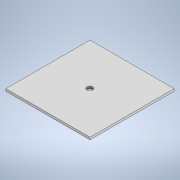
# Autodesk Inventor part: Base
Saved by Autodesk Inventor 2020 (Build 240168000, 168)
## iProperties
Created: 2019-09-27
Part Number: Base
Material: Genérico
Document SubType Name: Modeling
Designer: Java9
Density: 1 g/cm^3
Appearance: Valor por defecto
Author: Java9
Autodesk Inventor part; units mm, degrees
ref_plane "YZ Plane" through (0, 0, 0) normal (1, 0, 0) x (0, 1, 0)
ref_plane "XZ Plane" through (0, 0, 0) normal (0, 1, 0) x (-1, 0, 0)
ref_plane "XY Plane" through (0, 0, 0) normal (0, 0, 1) x (1, 0, 0)
sketch "Boceto1" plane through (0, 0, 0) normal (0, 0, 1) x (1, 0, 0)
  line L0 (0, 0) -> (450, 0)
  line L1 (450, 0) -> (450, 12.7)
  line L2 (450, 12.7) -> (0, 12.7)
  line L3 (0, 12.7) -> (0, 0)
  dimension "d0" = 450
  dimension "d1" = 12.7
  constraints: 8 end point, 2 perpendicular, 1 horizontal, 1 parallel
  measures "d0" distance of L0.start L0.end
  measures "d1" distance of L0.end L1.end
extrude "Extrusión1" add sketch "Boceto1" along normal blind 450
sketch "Boceto2" plane through (0, 12.7, 0) normal (0, 1, 0) x (1, 0, 0)
  line L0 (0, -450) -> (450, -450) projected
  circle A0 centre (224.0346, -225.001) radius 10
  point P0 (0, 0)
  dimension "d4" = 20
  constraints: 1 centre point
  measures "d4" diameter of A0
hole "Agujero1" at (224.0346, 12.7, 225.001) direction (0, -1, 0) diameter 30 end through all
